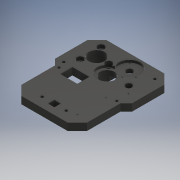
# Autodesk Inventor part: AC02
Saved by Autodesk Inventor 2017 (Build 210142000, 142)
## iProperties
Created: 2019-08-28
Part Number: AC02
Material: ABS Plastic
Document SubType Name: Modeling
Designer: Dell
Density: 1.06 g/cm^3
Appearance: Smooth - Black
Author: Dell
Autodesk Inventor part; units mm, degrees
ref_plane "YZ Plane" through (0, 0, 0) normal (1, 0, 0) x (0, 1, 0)
ref_plane "XZ Plane" through (0, 0, 0) normal (0, 1, 0) x (-1, 0, 0)
ref_plane "XY Plane" through (0, 0, 0) normal (0, 0, 1) x (1, 0, 0)
sketch "Sketch35" plane through (0, 0, 0) normal (0, 0, 1) x (1, 0, 0)
  line L0 (0, 86.6025) -> (75, 43.3013)
  line L1 (75, 43.3013) -> (75, -43.3013)
  line L2 (75, -43.3013) -> (0, -86.6025)
  line L3 (0, -86.6025) -> (-75, -43.3013)
  line L4 (-75, -43.3013) -> (-75, 43.3013)
  line L5 (-75, 43.3013) -> (0, 86.6025)
  line L6 (-75, -43.3013) -> (-75, -130)
  line L7 (-75, -130) -> (75, -130)
  line L8 (75, -130) -> (75, -43.3013)
  point P0 (0, 0)
  point P1 (0, 0)
  dimension "d165" = 150
  dimension "d166" = 130
  constraints: 18 end point, 2 perpendicular, 1 coincident, 1 vertical, 1 vertical alignment, 13 other
  measures "d165" distance between parallel lines of L1 L4
  measures "d166" distance from line of L7 point (0, 0)
extrude "Extrusion34" add sketch "Sketch35" along normal blind 55
sketch "Sketch36" plane through (0, 0, 55) normal (0, 0, 1) x (1, 0, 0)
  line L0 (75, -130) -> (75, 43.3013) construction
  line L1 (75, 43.3013) -> (0, 86.6025) construction
  line L2 (0, 86.6025) -> (-75, 43.3013) construction
  line L3 (-75, 43.3013) -> (-75, -130) construction
  line L4 (-75, -130) -> (75, -130) construction
  line L5 (68, 39.2598) -> (68, -123) construction
  line L6 (68, -123) -> (-68, -123) construction
  line L7 (-68, -123) -> (-68, 39.2598) construction
  line L8 (-68, 39.2598) -> (0, 78.5196) construction
  line L9 (0, 78.5196) -> (68, 39.2598) construction
  circle A0 centre (-68, -123) radius 2
  circle A1 centre (68, -123) radius 2
  circle A2 centre (0, 78.5196) radius 2
  circle A3 centre (-68, 39.2598) radius 2
  circle A4 centre (68, 39.2598) radius 2
  circle A5 centre (-34, -123) radius 2
  circle A6 centre (34, -123) radius 2
  circle A7 centre (0, -123) radius 2
  circle A8 centre (-68, -71.8701) radius 2
  circle A9 centre (-68, -41.8701) radius 2
  circle A10 centre (-68, 0) radius 2
  circle A11 centre (68, 0) radius 2
  circle A12 centre (68, -41.8701) radius 2
  circle A13 centre (68, -71.8701) radius 2
  circle A14 centre (-34, 58.8897) radius 2
  circle A15 centre (34, 58.8897) radius 2
  point P0 (0, 0)
  dimension "d169" = 7
  dimension "d170" = 4
  dimension "d171" = 4
  dimension "d172" = 4
  dimension "d173" = 4
  dimension "d174" = 4
  dimension "d175" = 4
  dimension "d176" = 4
  dimension "d177" = 4
  dimension "d178" = 4
  dimension "d179" = 4
  dimension "d180" = 4
  dimension "d181" = 4
  dimension "d182" = 4
  dimension "d183" = 4
  dimension "d184" = 4
  dimension "d185" = 4
  dimension "d186" = 30
  constraints: 16 centre point, 10 end point, 6 point on line, 5 coincident, 5 midpoint, 3 horizontal alignment, 2 vertical alignment, 4 other
  measures "d169" distance between parallel lines of L0 L5
  measures "d170" diameter of A0
  measures "d171" diameter of A1
  measures "d172" diameter of A2
  measures "d173" diameter of A3
  measures "d174" diameter of A4
  measures "d175" diameter of A5
  measures "d176" diameter of A6
  measures "d177" diameter of A7
  measures "d178" diameter of A8
  measures "d179" diameter of A9
  measures "d180" diameter of A10
  measures "d181" diameter of A11
  measures "d182" diameter of A12
  measures "d183" diameter of A13
  measures "d184" diameter of A14
  measures "d185" diameter of A15
  measures "d186" distance of A9.centre A8.centre
extrude "Extrusion35" cut sketch "Sketch36" against normal through all contours A0 | A1 | A3 | A4 | A9 | A12 | A14 | A15
sketch "Sketch37" plane through (0, 0, 55) normal (0, 0, 1) x (1, 0, 0)
  circle A0 centre (0, 0) radius 15
  dimension "d189" = 30
  constraints: 1 centre point, 1 coincident
  measures "d189" diameter of A0
extrude "Extrusion36" cut sketch "Sketch37" against normal blind 7
sketch "Sketch41" plane through (0, 0, 0) normal (0, 0, -1) x (-1, 0, 0)
  circle A0 centre (34, 58.8897) radius 2 projected
  circle A1 centre (-68, -41.8701) radius 2 projected
  circle A2 centre (-68, 39.2598) radius 2 projected
  circle A3 centre (68, -123) radius 2 projected
  circle A4 centre (-68, -123) radius 2 projected
  circle A5 centre (68, 39.2598) radius 2 projected
  circle A6 centre (68, -41.8701) radius 2 projected
  circle A7 centre (-34, 58.8897) radius 2 projected
  line L0 (-75, -130) -> (-75, 43.3013) projected
  line L1 (75, -130) -> (-75, -130) projected
  line L2 (75, 43.3013) -> (75, -130) projected
  line L3 (0, 86.6025) -> (75, 43.3013) projected
  line L4 (-75, 43.3013) -> (0, 86.6025) projected
  line L5 (0, 70.4367) -> (61, 35.2184)
  line L6 (61, 35.2184) -> (61, -116)
  line L7 (61, -116) -> (-61, -116)
  line L8 (-61, -116) -> (-61, 35.2184)
  line L9 (-61, 35.2184) -> (0, 70.4367)
  point P0 (0, 0)
  dimension "d199" = 14
  constraints: 10 end point, 4 other
  measures "d199" distance between parallel lines of L8 L0
extrude "Extrusion39" cut sketch "Sketch41" against normal blind 40 contours L0 L4 L3 L2 L1 | L5 L6 L7 L8 L9
sketch "Sketch42" plane through (0, 0, 40) normal (0, 0, -1) x (-1, 0, 0)
  circle A0 centre (0, 0) radius 7.5
  circle A1 centre (-45, 0) radius 4
  circle A2 centre (-14.7916, 31.7208) radius 4
  circle A3 centre (40.7839, 19.0178) radius 4
  line L0 (0, 0) -> (32.276, 0) construction
  line L1 (0, 0) -> (-45, 0) construction
  line L2 (0, 0) -> (-14.7916, 31.7208) construction
  circle A4 centre (15.7839, 19.0178) radius 3.5
  circle A5 centre (53.2839, -2.6328) radius 3.5
  circle A6 centre (53.2839, 40.6685) radius 3.5
  line L3 (0, 0) -> (40.7839, 19.0178) construction
  dimension "d202" = 15
  dimension "d203" = 8
  dimension "d204" = 8
  dimension "d205" = 8
  dimension "d206" = 45
  dimension "d207" = 35
  dimension "d208" = 45
  dimension "d219" = 180
  dimension "d220" = 115
  dimension "d298" = 7
  dimension "d299" = 25
  dimension "d302" = 360
  dimension "d304" = 25
  constraints: 8 end point, 7 centre point, 1 coincident, 1 horizontal, 1 vertical alignment, 7 other
  measures "d202" diameter of A0
  measures "d203" diameter of A1
  measures "d204" diameter of A2
  measures "d205" diameter of A3
  measures "d206" distance of point (0, 0) L3.end
  measures "d207" distance of point (0, 0) L2.end
  measures "d208" distance of point (0, 0) L1.end
  measures "d219" angle of L0 L1
  measures "d220" angle of L2 L0
  measures "d298" diameter of A4
  measures "d299" distance of L3.end A4.centre
  measures "d304" angle of L0 L3
extrude "Extrusion40" cut sketch "Sketch42" against normal through all
sketch "Sketch43" plane through (0, 0, 40) normal (0, 0, -1) x (-1, 0, 0)
  line L0 (-6.5, -103) -> (6.5, -103)
  line L1 (6.5, -103) -> (6.5, -116)
  line L2 (6.5, -116) -> (-6.5, -116)
  line L3 (-6.5, -116) -> (-6.5, -103)
  line L4 (75, -130) -> (-75, -130) projected
  point P0 (0, 0)
  point P1 (0, -103)
  dimension "d221" = 13
  dimension "d222" = 13
  dimension "d223" = 27
  constraints: 8 end point, 2 parallel, 1 horizontal, 1 midpoint, 1 perpendicular, 1 vertical alignment
  measures "d221" distance of L1.end L2.end
  measures "d222" distance of L0.end L1.end
  measures "d223" distance between parallel lines of L4 L0
extrude "Extrusion41" cut sketch "Sketch43" against normal through all
sketch "Sketch44" plane through (0, 0, 40) normal (0, 0, -1) x (-1, 0, 0)
  circle A0 centre (0, 71.6025) radius 2
  circle A1 centre (-50, -105) radius 2
  line L0 (-75, -130) -> (-75, 43.3013) projected
  line L1 (75, -130) -> (-75, -130) projected
  point P0 (0, 0)
  point P1 (0, 86.6025)
  dimension "d226" = 4
  dimension "d227" = 4
  dimension "d228" = 15
  dimension "d229" = 25
  dimension "d230" = 25
  constraints: 2 centre point, 1 vertical alignment
  measures "d226" diameter of A0
  measures "d227" diameter of A1
  measures "d228" distance of point (0, 86.603) A0.centre
  measures "d229" distance from line of L0 A1.centre
  measures "d230" distance from line of L1 A1.centre
extrude "Extrusion42" cut sketch "Sketch44" against normal through all
sketch "Sketch53" plane through (0, 0, 55) normal (0, 0, 1) x (1, 0, 0)
  circle A0 centre (14.7916, 31.7208) radius 4 projected
  circle A1 centre (14.7916, 31.7208) radius 10
  circle A2 centre (45, 0) radius 4 projected
  circle A3 centre (45, 0) radius 10
  point P0 (0, 0)
  dimension "d261" = 20
  dimension "d262" = 20
  constraints: 2 centre point, 2 coincident
  measures "d261" diameter of A1
  measures "d262" diameter of A3
extrude "Extrusion49" cut sketch "Sketch53" against normal blind 6
sketch "Sketch54" plane through (0, 0, 40) normal (0, 0, -1) x (-1, 0, 0)
  circle A0 centre (-14.7916, 31.7208) radius 4 projected
  circle A1 centre (-14.7916, 31.7208) radius 10
  circle A2 centre (-45, 0) radius 4 projected
  circle A3 centre (-45, 0) radius 10
  point P0 (0, 0)
  dimension "d265" = 20
  dimension "d266" = 20
  constraints: 2 centre point, 2 coincident
  measures "d265" diameter of A1
  measures "d266" diameter of A3
extrude "Extrusion50" cut sketch "Sketch54" against normal blind 6
sketch "Sketch56" plane through (0, 0, 40) normal (0, 0, -1) x (-1, 0, 0)
  line L0 (-28.3863, 25.3815) -> (-1.197, 38.06) construction
  line L1 (0, 0) -> (-14.7916, 31.7208) construction
  circle A0 centre (-45, 0) radius 4 construction
  line L2 (0, 0) -> (-45, 0) construction
  line L3 (-45, 15) -> (-45, -15) construction
  circle A1 centre (-14.7916, 31.7208) radius 4 construction
  circle A2 centre (-1.197, 38.06) radius 0.75
  circle A3 centre (-28.3863, 25.3815) radius 0.75
  circle A4 centre (-45, 15) radius 0.75
  circle A5 centre (-45, -15) radius 0.75
  dimension "d272" = 30
  dimension "d273" = 30
  dimension "d274" = 1.5
  dimension "d275" = 1.5
  dimension "d276" = 1.5
  dimension "d277" = 1.5
  constraints: 8 end point, 5 coincident, 4 centre point, 2 midpoint, 2 perpendicular
  measures "d272" distance of L0.start L0.end
  measures "d273" distance of L3.start L3.end
  measures "d274" diameter of A2
  measures "d275" diameter of A3
  measures "d276" diameter of A4
  measures "d277" diameter of A5
extrude "Extrusion51" cut sketch "Sketch56" against normal through all
sketch "Sketch58" plane through (0, 0, 40) normal (0, 0, -1) x (-1, 0, 0)
  circle A0 centre (-35, -75) radius 0.75
  circle A1 centre (-10, -50) radius 0.75
  point P0 (0, 0)
  dimension "d286" = 1.5
  dimension "d287" = 1.5
  dimension "d288" = 50
  dimension "d289" = 10
  dimension "d290" = 25
  dimension "d291" = 25
  constraints: 2 centre point
  measures "d286" diameter of A0
  measures "d287" diameter of A1
  measures "d288" vertical distance of point (0, 0) A1.centre
  measures "d289" horizontal distance of A1.centre point (0, 0)
  measures "d290" horizontal distance of A1.centre A0.centre
  measures "d291" horizontal distance of A1.centre A0.centre
extrude "Extrusion53" cut sketch "Sketch58" against normal through all
sketch "Sketch60" plane through (0, 0, 40) normal (0, 0, -1) x (-1, 0, 0)
  line L0 (68.1273, -110) -> (48.1273, -130) construction
  line L1 (68.1273, -40) -> (68.1273, -110) construction
  line L2 (80.1273, -28) -> (68.1273, -40) construction
  line L3 (80.1273, 39) -> (80.1273, -28) construction
  line L4 (60.1273, 59) -> (80.1273, 39) construction
  line L5 (-60.1273, 59) -> (60.1273, 59) construction
  line L6 (-80.1273, 39) -> (-60.1273, 59) construction
  line L7 (-80.1273, -28) -> (-80.1273, 39) construction
  line L8 (-68.1273, -40) -> (-80.1273, -28) construction
  line L9 (-68.1273, -40) -> (-68.1273, -110) construction
  line L10 (-48.1273, -130) -> (-68.1273, -110) construction
  line L11 (-48.1273, -130) -> (-37.5219, -130) construction
  line L12 (-37.5219, -130) -> (37.5219, -130) construction
  line L13 (37.5219, -130) -> (48.1273, -130) construction
  line L14 (-48.1273, -130) -> (48.1273, -130) construction
  line L15 (75, -130) -> (-75, -130) construction
  circle A0 centre (-35, -75) radius 0.75 construction
  circle A1 centre (-10, -50) radius 0.75 construction
  circle A2 centre (-45, 15) radius 0.75 construction
  circle A3 centre (-1.197, 38.06) radius 0.75 construction
  circle A4 centre (-28.3863, 25.3815) radius 0.75 construction
  circle A5 centre (-45, -15) radius 0.75 construction
  circle A6 centre (-14.7916, 31.7208) radius 10 construction
  circle A7 centre (-45, 0) radius 10 construction
  circle A8 centre (0, 71.6025) radius 2 construction
  circle A9 centre (-50, -105) radius 2 construction
  line L16 (-6.5, -116) -> (-6.5, -103) construction
  line L17 (-6.5, -103) -> (6.5, -103) construction
  line L18 (6.5, -103) -> (6.5, -116) construction
  line L19 (6.5, -116) -> (-6.5, -116) construction
  circle A10 centre (40.7839, 19.0178) radius 4 construction
  circle A11 centre (53.2839, -2.6328) radius 3.5 construction
  circle A12 centre (15.7839, 19.0178) radius 3.5 construction
  circle A13 centre (53.2839, 40.6685) radius 3.5 construction
  circle A14 centre (0, 0) radius 7.5 construction
  circle A15 centre (-34, 58.8897) radius 2 construction
  circle A16 centre (68, -41.8701) radius 2 construction
  circle A17 centre (68, 39.2598) radius 2 construction
  circle A18 centre (-68, -123) radius 2 construction
  circle A19 centre (68, -123) radius 2 construction
  circle A20 centre (-68, 39.2598) radius 2 construction
  circle A21 centre (-68, -41.8701) radius 2 construction
  circle A22 centre (34, 58.8897) radius 2 construction
  line L20 (-75, -130) -> (-75, 43.3013) construction
  line L21 (75, -130) -> (-75, -130) construction
  line L22 (75, 43.3013) -> (75, -130) construction
  line L23 (0, 86.6025) -> (75, 43.3013) construction
  line L24 (-75, 43.3013) -> (0, 86.6025) construction
  line L25 (-60.1273, 59) -> (-47.809, 59)
  line L26 (-75, 43.3013) -> (0, 86.6025) projected
  line L27 (-47.809, 59) -> (-75, 43.3013)
  line L28 (-75, 43.3013) -> (-75, -33.1273)
  line L29 (-75, -33.1273) -> (-80.1273, -28)
  line L30 (-80.1273, -28) -> (-80.1273, 39)
  line L31 (-80.1273, 39) -> (-60.1273, 59)
  line L32 (-75, -33.1273) -> (-68.1273, -40)
  line L33 (-68.1273, -40) -> (-68.1273, -110)
  line L34 (-48.1273, -130) -> (-68.1273, -110)
  line L35 (75, -130) -> (-75, -130) projected
  line L36 (-48.1273, -130) -> (-75, -130)
  line L37 (-75, -130) -> (-75, -33.1273)
  line L38 (-47.809, 59) -> (0, 86.6025)
  line L39 (0, 86.6025) -> (0, 59)
  line L40 (0, 59) -> (-47.809, 59)
  point P0 (0, -130)
  point P1 (0, -130)
  dimension "d305" = 67
  dimension "d306" = 120.2547
  dimension "d308" = 20
  dimension "d309" = 12
  dimension "d310" = 12
  dimension "d311" = 70
  dimension "d312" = 20
  dimension "d313" = 20
  dimension "d314" = 96.2547
  dimension "d315" = 20
  dimension "d316" = 20
  dimension "d317" = 20
  dimension "d318" = 135
  dimension "d319" = 135
  dimension "d320" = 135
  dimension "d321" = 135
  dimension "d322" = 12
  dimension "d323" = 12
  dimension "d324" = 67
  dimension "d325" = 70
  dimension "d326" = 20
  dimension "d327" = 20
  dimension "d328" = 135
  constraints: 58 end point, 7 collinear, 5 point on line, 3 midpoint, 2 horizontal, 2 vertical alignment, 1 perpendicular
  measures "d305" distance of L8.end L7.end
  measures "d306" distance of L5.start L4.start
  measures "d308" distance from line of L7.end L5
  measures "d309" horizontal distance of L9.start L8.end
  measures "d310" horizontal distance of L9.start L8.end
  measures "d311" distance of L9.start L9.end
  measures "d312" horizontal distance of L10.start L9.end
  measures "d313" horizontal distance of L10.start L9.end
  measures "d314" distance of L13.end L10.start
  measures "d315" horizontal distance of L4.start L3.start
  measures "d316" horizontal distance of L4.start L3.start
  measures "d317" horizontal distance of L7.end L5.start
  measures "d318" angle of L7 L6
  measures "d319" angle of L5 L6
  measures "d320" angle of L9 L8
  measures "d321" angle of L10 L11
  measures "d322" horizontal distance of L2.start L1.start
  measures "d323" horizontal distance of L2.start L1.start
  measures "d324" distance of L3.start L2.start
  measures "d325" distance of L1.start L1.end
  measures "d326" horizontal distance of L1.end L13.end
  measures "d327" horizontal distance of L1.end L13.end
  measures "d328" angle of L0 L1
extrude "Extrusion55" add sketch "Sketch60" against normal up to surface (15 mm away) from surface at 0 contours L25 L26 L28 L29 L30 L31
mirror "Mirror1" about plane through (0, 0, 0) normal (1, 0, 0) of "Extrusion55"
extrude "Extrusion56" cut sketch "Sketch60" against normal through all contours L26 L39 L40 | L32 L33 L34 L35 L37
mirror "Mirror2" about plane through (0, 0, 0) normal (1, 0, 0) of "Extrusion56"
sketch "Sketch61" plane through (0, 0, 40) normal (0, 0, -1) x (-1, 0, 0)
  circle A0 centre (-68, 39.2598) radius 2 projected
  circle A1 centre (68, 39.2598) radius 2 projected
  arc A2 (32.003, 59) -> (35.997, 59) centre (34, 58.8897) ccw projected
  arc A3 (-35.997, 59) -> (-32.003, 59) centre (-34, 58.8897) ccw projected
  arc A4 (-68.1273, -43.866) -> (-68.2425, -39.8848) centre (-68, -41.8701) ccw projected
  arc A5 (68.2425, -39.8848) -> (68.1273, -43.866) centre (68, -41.8701) ccw projected
  circle A6 centre (-50, -105) radius 2 projected
  circle A7 centre (-35, -75) radius 0.75 projected
  circle A8 centre (-10, -50) radius 0.75 projected
  line L0 (-35.997, 59) -> (-32.003, 59)
  line L1 (60.1273, 59) -> (35.997, 59) projected
  line L2 (32.003, 59) -> (35.997, 59)
  arc A9 (68.2425, -39.8848) -> (68.1273, -43.866) centre (68, -41.8701) ccw projected
  line L3 (68.2425, -39.8848) -> (68.1273, -40)
  line L4 (68.1273, -40) -> (68.1273, -43.866)
  line L5 (68.1273, -110) -> (68.1273, -43.866) projected
  line L6 (68.2425, -39.8848) -> (80.1273, -28) projected
  line L7 (-68.2425, -39.8848) -> (-68.1273, -40)
  line L8 (-68.1273, -43.866) -> (-68.1273, -110) projected
  line L9 (-68.1273, -40) -> (-68.1273, -43.866)
  line L10 (-80.1273, -28) -> (-68.2425, -39.8848) projected
  point P0 (0, 0)
  constraints: 12 end point, 5 collinear, 1 horizontal
extrude "Extrusion57" add sketch "Sketch61" against normal up to surface (15 mm away) from surface at 0
sketch "Sketch62" plane through (0, 0, 40) normal (0, 0, -1) x (-1, 0, 0)
  circle A0 centre (40.7839, 19.0178) radius 4 projected
  circle A1 centre (40.7839, 19.0178) radius 16.5
  point P0 (0, 0)
  dimension "d335" = 33
  constraints: 1 centre point, 1 coincident
  measures "d335" diameter of A1
extrude "Extrusion58" cut sketch "Sketch62" against normal through all
sketch "Sketch63" plane through (0, 0, 55) normal (0, 0, 1) x (1, 0, 0)
  circle A0 centre (-15.7839, 19.0178) radius 3.5 projected
  circle A1 centre (-15.7839, 19.0178) radius 7
  circle A2 centre (-40.7839, 19.0178) radius 16.5 projected
  circle A3 centre (-53.2839, 40.6685) radius 7
  circle A4 centre (-53.2839, -2.6328) radius 7
  point P0 (0, 0)
  dimension "d338" = 14
  dimension "d341" = 360
  constraints: 3 centre point, 1 coincident, 7 other
  measures "d338" diameter of A1
extrude "Extrusion59" cut sketch "Sketch63" against normal up to surface (7 mm away) from surface at 0 contours A0 | A1 | A2 | A3 | A4
sketch "Sketch64" plane through (0, 0, 40) normal (0, 0, -1) x (-1, 0, 0)
  circle A0 centre (15.7839, 19.0178) radius 3.5 projected
  circle A1 centre (53.2839, 40.6685) radius 3.5 projected
  circle A2 centre (53.2839, -2.6328) radius 3.5 projected
  circle A3 centre (15.7839, 19.0178) radius 3.5 projected
  circle A4 centre (15.7839, 19.0178) radius 8
  circle A5 centre (40.7839, 19.0178) radius 16.5 construction
  circle A6 centre (53.2839, -2.6328) radius 8
  circle A7 centre (53.2839, 40.6685) radius 8
  point P0 (0, 0)
  dimension "d345" = 16
  dimension "d348" = 360
  constraints: 3 centre point, 1 coincident, 7 other
  measures "d345" diameter of A4
extrude "Extrusion60" add sketch "Sketch64" along normal blind 10
sketch "Sketch65" plane through (0, 0, 55) normal (0, 0, 1) x (1, 0, 0)
  line L0 (-25, -110) -> (25, -110)
  line L1 (-48.1273, -130) -> (48.1273, -130) projected
  circle A0 centre (-25, -110) radius 2.75
  circle A1 centre (25, -110) radius 2.75
  point P0 (0, 0)
  point P1 (0, -110)
  dimension "d352" = 20
  dimension "d353" = 50
  dimension "d354" = 5.5
  dimension "d355" = 5.5
  constraints: 2 centre point, 2 coincident, 2 end point, 1 horizontal, 1 midpoint, 1 vertical alignment
  measures "d352" distance between parallel lines of L1 L0
  measures "d353" distance of L0.start L0.end
  measures "d354" diameter of A0
  measures "d355" diameter of A1
extrude "Extrusion61" cut sketch "Sketch65" against normal through all
sketch "Sketch66" plane through (0, 0, 40) normal (0, 0, -1) x (-1, 0, 0)
  circle A0 centre (-60.1273, 39) radius 2.75
  line L0 (60.1273, 59) -> (-60.1273, 59) projected
  line L1 (-80.1273, 39) -> (-80.1273, -28) projected
  circle A1 centre (65.1273, -25) radius 2.75
  line L2 (80.1273, 39) -> (80.1273, -28) projected
  point P0 (0, 0)
  point P1 (68.1273, -40)
  dimension "d358" = 5.5
  dimension "d359" = 20
  dimension "d360" = 20
  dimension "d361" = 5.5
  dimension "d362" = 15
  dimension "d363" = 15
  constraints: 2 centre point
  measures "d358" diameter of A0
  measures "d359" distance from line of L0 A0.centre
  measures "d360" distance from line of L1 A0.centre
  measures "d361" diameter of A1
  measures "d362" distance from line of L2 A1.centre
  measures "d363" vertical distance of A1.centre point (68.127, -40)
extrude "Extrusion62" cut sketch "Sketch66" against normal through all
sketch "Sketch67" plane through (0, 0, 40) normal (0, 0, -1) x (-1, 0, 0)
  circle A0 centre (40.7839, 19.0178) radius 16.5 projected
  circle A1 centre (40.7839, 19.0178) radius 17
  circle A2 centre (15.7839, 19.0178) radius 8 projected
  circle A3 centre (40.7839, 19.0178) radius 33
  circle A4 centre (15.7839, 19.0178) radius 8 projected
  circle A5 centre (53.2839, 40.6685) radius 3.5 projected
  circle A6 centre (53.2839, -2.6328) radius 3.5 projected
  point P0 (0, 0)
  constraints: 2 centre point, 2 coincident, 2 tangent
extrude "Extrusion63" add sketch "Sketch67" along normal blind 10 contours A1 | A3
sketch "Sketch68" plane through (0, 0, 55) normal (0, 0, 1) x (1, 0, 0)
  line L0 (-60, -40) -> (60, -40) construction
  line L1 (-48.1273, -130) -> (48.1273, -130) projected
  circle A0 centre (-60, -40) radius 2.5
  circle A1 centre (60, -40) radius 2.5
  point P0 (0, 0)
  point P1 (0, -40)
  dimension "d368" = 90
  dimension "d369" = 120
  dimension "d370" = 5
  dimension "d371" = 5
  constraints: 2 centre point, 2 coincident, 2 end point, 1 horizontal, 1 midpoint, 1 vertical alignment
  measures "d368" distance between parallel lines of L1 L0
  measures "d369" distance of L0.start L0.end
  measures "d370" diameter of A0
  measures "d371" diameter of A1
extrude "Extrusion64" cut sketch "Sketch68" against normal through all
sketch "Sketch69" plane through (0, 0, 55) normal (0, 0, 1) x (1, 0, 0)
  circle A0 centre (43.1273, -45) radius 1
  circle A1 centre (43.1273, -105) radius 1
  line L0 (-48.1273, -130) -> (48.1273, -130) projected
  line L1 (-68.1273, -110) -> (-68.1273, -40) projected
  line L2 (68.1273, -40) -> (68.1273, -110) projected
  point P0 (0, 0)
  dimension "d376" = 2
  dimension "d377" = 2
  dimension "d379" = 60
  dimension "d380" = 25
  dimension "d384" = 25
  constraints: 2 centre point, 1 vertical alignment
  measures "d376" diameter of A0
  measures "d377" diameter of A1
  measures "d379" distance of A1.centre A0.centre
  measures "d380" distance from line of L0 A1.centre
  measures "d384" distance from line of L2 A1.centre
extrude "Extrusion65" cut sketch "Sketch69" against normal through all
sketch "Sketch71" plane through (0, 0, 40) normal (0, 0, -1) x (-1, 0, 0)
  circle A0 centre (-28.3863, 25.3815) radius 0.75 projected
  circle A1 centre (-14.7916, 31.7208) radius 4 projected
  circle A2 centre (-14.7916, 31.7208) radius 10 projected
  circle A3 centre (-1.197, 38.06) radius 0.75 projected
  circle A4 centre (-45, 15) radius 0.75 projected
  circle A5 centre (-45, 0) radius 4 projected
  circle A6 centre (-45, 0) radius 10 projected
  circle A7 centre (-45, -15) radius 0.75 projected
  point P0 (0, 0)
extrude "Extrusion66" add sketch "Sketch71" against normal up to surface (15 mm away) from surface at 0
sketch "Sketch72" plane through (0, 0, 40) normal (0, 0, -1) x (-1, 0, 0)
  circle A0 centre (-14.7916, 31.7208) radius 4 projected
  circle A1 centre (-14.7916, 31.7208) radius 16.25
  circle A2 centre (-45, 0) radius 4 projected
  circle A3 centre (-45, 0) radius 16.25
  point P0 (0, 0)
  dimension "d388" = 32.5
  dimension "d389" = 32.5
  constraints: 2 centre point, 2 coincident
  measures "d388" diameter of A1
  measures "d389" diameter of A3
extrude "Extrusion67" cut sketch "Sketch72" against normal blind 5
sketch "Sketch73" plane through (0, 0, 40) normal (0, 0, -1) x (-1, 0, 0)
  circle A0 centre (-14.7916, 31.7208) radius 4 projected
  circle A1 centre (-14.7916, 31.7208) radius 6.5
  circle A2 centre (-45, 0) radius 6.5
  circle A3 centre (-45, 0) radius 4 projected
  point P0 (0, 0)
  dimension "d392" = 13
  dimension "d393" = 13
  constraints: 2 centre point, 2 coincident
  measures "d392" diameter of A1
  measures "d393" diameter of A2
extrude "Extrusion68" cut sketch "Sketch73" along normal through all both and the other way through all contours A0 | A1 | A2 | A3
sketch "Sketch74" plane through (0, 0, 55) normal (0, 0, 1) x (1, 0, 0)
  circle A0 centre (0, 0) radius 15 projected
extrude "Extrusion69" cut sketch "Sketch74" against normal through all
sketch "Sketch75" plane through (0, 0, 55) normal (0, 0, 1) x (1, 0, 0)
  circle A0 centre (0, 0) radius 21
  circle A1 centre (14.7916, 31.7208) radius 6.5 projected
  circle A2 centre (14.7916, 31.7208) radius 22
  dimension "d398" = 42
  dimension "d399" = 44
  constraints: 2 centre point, 2 coincident
  measures "d398" diameter of A0
  measures "d399" diameter of A2
extrude "Extrusion70" cut sketch "Sketch75" against normal blind 5
sketch "Sketch76" plane through (-15.7839, 19.0178, 48) normal (0, 0, 1) x (1, 0, 0)
  circle A0 centre (0, 0) radius 3.5 projected
  circle A1 centre (0, 0) radius 7 projected
  point P0 (15.7839, -19.0178)
extrude "Extrusion71" cut sketch "Sketch76" against normal blind 4
sketch "Sketch78" plane through (0, 0, 40) normal (0, 0, -1) x (-1, 0, 0)
  circle A0 centre (-14.7916, 31.7208) radius 6.5 projected
  circle A1 centre (-45, 0) radius 6.5 projected
  line L0 (1.5329, 48.8626) -> (-61.3245, -17.1418) construction
  line L1 (1.5329, 48.8626) -> (7.2379, 29.4774)
  line L2 (7.2379, 29.4774) -> (-6.6977, 14.8441)
  line L3 (-6.6977, 14.8441) -> (-26.3383, 19.5961) construction
  line L4 (-26.3383, 19.5961) -> (-32.0433, 38.9813) construction
  line L5 (-32.0433, 38.9813) -> (-18.1077, 53.6145)
  line L6 (-18.1077, 53.6145) -> (1.5329, 48.8626)
  line L7 (-61.3245, -17.1418) -> (-67.0295, 2.2434)
  line L8 (-67.0295, 2.2434) -> (-53.094, 16.8766)
  line L9 (-53.094, 16.8766) -> (-33.4534, 12.1247) construction
  line L10 (-33.4534, 12.1247) -> (-27.7484, -7.2605) construction
  line L11 (-27.7484, -7.2605) -> (-41.684, -21.8938)
  line L12 (-41.684, -21.8938) -> (-61.3245, -17.1418)
  line L13 (-32.0433, 38.9813) -> (-50.5659, 19.5313)
  line L14 (-6.6977, 14.8441) -> (-27.7484, -7.2605)
  line L15 (-14.7916, 31.7208) -> (-45, 0) construction
  circle A2 centre (-14.7916, 31.7208) radius 6.5 projected
  circle A3 centre (-14.7916, 31.7208) radius 16.25 projected
  circle A4 centre (-45, 0) radius 6.5 projected
  circle A5 centre (-45, 0) radius 16.25 projected
  line L16 (-67.0295, 2.2434) -> (-18.1077, 53.6145)
  line L17 (7.2379, 29.4774) -> (-41.684, -21.8938)
  point P0 (0, 0)
  point P1 (-12.4027, 34.2293)
  point P2 (-47.389, -2.5086)
  point P3 (-29.8958, 15.8604)
  dimension "d436" = 91.1463
  dimension "d437" = 35
  dimension "d438" = 35
  constraints: 37 end point, 5 point on line, 2 midpoint, 1 collinear, 1 parallel, 26 other
  measures "d436" distance of L0.end L0.start
  measures "d437" distance between parallel lines of L5 L2
  measures "d438" distance between parallel lines of L8 L11
extrude "Extrusion72" add sketch "Sketch78" along normal blind 5 contours L1 L2 L14 L11 L12 L7 L8 L16 L13 L5 L6
sketch "Sketch79" plane through (0, 0, 35) normal (0, 0, -1) x (-1, 0, 0)
  circle A0 centre (-14.7916, 31.7208) radius 6.5 projected
  circle A1 centre (-45, 0) radius 6.5 construction
  line L0 (-14.7916, 31.7208) -> (-45, 0) construction
  line L1 (-37.1374, 22.7567) -> (-22.6542, 8.9641) construction
  circle A2 centre (-22.6542, 8.9641) radius 1.05
  circle A3 centre (-37.1374, 22.7567) radius 1.05
  circle A4 centre (-0.536, 46.6901) radius 1.05
  circle A5 centre (-59.2556, -14.9694) radius 1.05
  line L2 (-18.1077, 53.6145) -> (1.5329, 48.8626) projected
  line L3 (-41.684, -21.8938) -> (-61.3245, -17.1418) projected
  line L4 (1.5329, 48.8626) -> (-61.3245, -17.1418) construction
  line L5 (-0.536, 46.6901) -> (-59.2556, -14.9694)
  point P0 (0, 0)
  point P1 (-29.8958, 15.8604)
  dimension "d441" = 20
  dimension "d442" = 2.1
  dimension "d443" = 2.1
  dimension "d444" = 2.1
  dimension "d445" = 2.1
  dimension "d452" = 85.1463
  constraints: 8 end point, 4 centre point, 4 midpoint, 2 coincident, 2 point on line, 1 collinear, 1 perpendicular
  measures "d441" distance of L1.start L1.end
  measures "d442" diameter of A2
  measures "d443" diameter of A3
  measures "d444" diameter of A4
  measures "d445" diameter of A5
  measures "d452" distance of L5.end L5.start
extrude "Extrusion73" cut sketch "Sketch79" against normal through all
sketch "Sketch80" plane through (0, 0, 40) normal (0, 0, -1) x (-1, 0, 0)
  circle A0 centre (-0.536, 46.6901) radius 1.05 projected
  circle A1 centre (-0.536, 46.6901) radius 4.4214
  circle A2 centre (-14.7916, 31.7208) radius 16.25 projected
  circle A3 centre (-59.2556, -14.9694) radius 1.05 projected
  circle A4 centre (-59.2556, -14.9694) radius 4.4214
  circle A5 centre (-45, 0) radius 16.25 projected
  circle A6 centre (-59.2556, -14.9694) radius 1.05 projected
  point P0 (0, 0)
  constraints: 2 centre point, 2 coincident, 2 tangent
extrude "Extrusion74" add sketch "Sketch80" along normal blind 5 contours A1 | A4
sketch "Sketch81" plane through (0, 0, 40) normal (0, 0, -1) x (-1, 0, 0)
  line L0 (47, -25) -> (12, -25)
  line L1 (12, -25) -> (12, -50)
  line L2 (12, -50) -> (47, -50)
  line L3 (47, -50) -> (47, -25)
  point P0 (0, 0)
  dimension "d455" = 25
  dimension "d456" = 35
  dimension "d457" = 25
  dimension "d458" = 12
  constraints: 8 end point, 2 parallel, 1 horizontal, 1 perpendicular
  measures "d455" distance of L2.end L0.start
  measures "d456" distance of L1.end L2.end
  measures "d457" distance from line of point (0, 0) L0
  measures "d458" distance from line of point (0, 0) L1
extrude "Extrusion75" cut sketch "Sketch81" against normal through all
body "Solid2"
